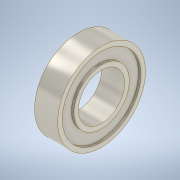
# Autodesk Inventor part: подшипник для ведущих шестеренок
Saved by Autodesk Inventor 2020.1 (Build 241239000, 239)
## iProperties
Created: 2021-12-18
Part Number: подшипник для ведущих шестеренок
Material: Титан
Document SubType Name: Modeling
Designer: Ni3na
Density: 4.51 g/cm^3
Appearance: Титан
Author: Ni3na
Autodesk Inventor part; units mm, degrees
ref_plane "YZ Plane" through (0, 0, 0) normal (1, 0, 0) x (0, 1, 0)
ref_plane "XZ Plane" through (0, 0, 0) normal (0, 1, 0) x (-1, 0, 0)
ref_plane "XY Plane" through (0, 0, 0) normal (0, 0, 1) x (1, 0, 0)
sketch "Эскиз6" plane through (0, 0, 0) normal (1, 0, 0) x (0, 1, 0)
  circle A0 centre (0, 0) radius 9.5
  circle A1 centre (0, 0) radius 5
  dimension "d13" = 19
  dimension "d14" = 10
  constraints: 2 centre point, 2 coincident
  measures "d13" diameter of A0
  measures "d14" diameter of A1
extrude "Выдавливание5" add sketch "Эскиз6" along normal blind 5
sketch "Эскиз7" plane through (5, 0, 0) normal (1, 0, 0) x (0, 0, -1)
  circle A0 centre (0, 0) radius 6
  circle A1 centre (0, 0) radius 8.5
  dimension "d17" = 12
  dimension "d18" = 17
  constraints: 2 centre point, 2 coincident
  measures "d17" diameter of A0
  measures "d18" diameter of A1
extrude "Выдавливание6" cut sketch "Эскиз7" against normal blind 0.5
sketch "Эскиз8" plane through (0, 0, 0) normal (-1, 0, 0) x (0, 0, 1)
  circle A0 centre (0, 0) radius 6
  circle A1 centre (0, 0) radius 8.4142
  constraints: 2 centre point, 2 coincident
extrude "Выдавливание7" cut sketch "Эскиз8" against normal blind 0.5
